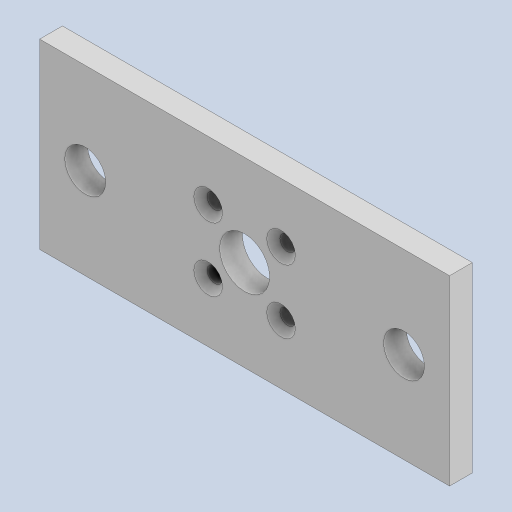
# Autodesk Inventor part: Al block2
Saved by Autodesk Inventor 2023.4 (Build 274418000, 418)
## iProperties
Created: 2024-01-11
Part Number: Al block2
Material: Generic
Document SubType Name: Modeling
Designer: PalumaCMM
Density: 1 g/cm^3
Appearance: Default
Author: PalumaCMM
Autodesk Inventor part; units mm, degrees
ref_plane "YZ Plane" through (0, 0, 0) normal (1, 0, 0) x (0, 1, 0)
ref_plane "XZ Plane" through (0, 0, 0) normal (0, 1, 0) x (-1, 0, 0)
ref_plane "XY Plane" through (0, 0, 0) normal (0, 0, 1) x (1, 0, 0)
sketch "Sketch1" plane through (0, 0, 0) normal (0, 0, 1) x (1, 0, 0)
  line L0 (0, 0) -> (60, 0)
  line L1 (60, 0) -> (60, 40)
  line L2 (60, 40) -> (0, 40)
  line L3 (0, 40) -> (0, 0)
  dimension "d0" = 60
  dimension "d1" = 40
  constraints: 8 end point, 2 parallel, 1 horizontal, 1 perpendicular
  measures "d0" distance of L2.end L1.end
  measures "d1" distance of L1.end L0.end
extrude "Extrusion1" add sketch "Sketch1" along normal blind 5
sketch "Sketch6" plane through (0, 0, 5) normal (0, 0, 1) x (1, 0, 0)
  point P0 (0, 0)
  point P1 (30, 20)
hole "Hole2" at (30, 20, 5) direction (0, 0, -1) diameter 11 end through all clearance for "Countersunk Flat Head Screw ISO 2009/7046" size "M10" standard "ISO"
sketch "Sketch7" plane through (0, 0, 5) normal (0, 0, 1) x (1, 0, 0)
  line L0 (0, 40) -> (0, 0) projected
  line L1 (60, 0) -> (60, 40) projected
  line L2 (60, 0) -> (0, 0)
  line L3 (60, 40) -> (0, 40) projected
  line L4 (30, 40) -> (30, 0)
  line L5 (0, 0) -> (60, 0) projected
  line L6 (0, 40) -> (0, 0) projected
  line L7 (0, 40) -> (-15, 40)
  line L8 (-15, 40) -> (-15, 0)
  line L9 (-15, 0) -> (0, 0)
  line L10 (0, 0) -> (0, 40)
  line L11 (60, 40) -> (60, 0)
  line L12 (60, 40) -> (60, 0)
  line L13 (60, 40) -> (75, 40)
  line L14 (75, 40) -> (75, 0)
  line L15 (75, 0) -> (60, 0)
  line L16 (0, 40) -> (-15, 40)
  point P0 (60, 0)
  point P1 (0, 0)
  dimension "d54" = 15
  dimension "d55" = 40
  constraints: 24 end point, 4 symmetric about line, 3 equal length, 2 midpoint, 2 point on line, 1 horizontal, 1 perpendicular
  measures "d54" distance of L9.end L8.end
  measures "d55" distance of L8.end L7.end
extrude "Extrusion3" add sketch "Sketch7" against normal blind 5 contours L0 L9 L8 L7 | L13 L14 L15 L1
sketch "Sketch9" plane through (0, 0, 5) normal (0, 0, 1) x (1, 0, 0)
  point P0 (0, 0)
  point P1 (-5, 20)
  point P2 (65, 20)
hole "Hole4" at (-5, 20, 5) at (65, 20, 5) direction (0, 0, -1) diameter 9 end through all clearance for "Countersunk Flat Head Screw ISO 2009/7046" size "M8" standard "ISO"
sketch "Sketch10" plane through (0, 0, 5) normal (0, 0, 1) x (1, 0, 0)
  line L0 (35.5, 14.5) -> (35.5, 25.5)
  line L1 (35.5, 14.5) -> (35.5, 25.5)
  line L2 (24.5, 25.5) -> (24.5, 14.5)
  line L3 (24.5, 25.5) -> (24.5, 14.5)
  line L4 (24.5, 14.5) -> (35.5, 25.5) construction
  line L5 (35.5, 14.5) -> (24.5, 25.5) construction
  circle A0 centre (30, 20) radius 5.5 projected
  line L6 (24.5, 30) -> (24.5, 10)
  line L7 (24.5, 10) -> (19.5, 10)
  line L8 (19.5, 10) -> (19.5, 30)
  line L9 (19.5, 30) -> (24.5, 30)
  line L10 (24.5, 20) -> (35.5, 20)
  line L11 (35.5, 30) -> (35.5, 10)
  line L12 (35.5, 10) -> (40.5, 10)
  line L13 (40.5, 10) -> (40.5, 30)
  line L14 (40.5, 30) -> (35.5, 30)
  point P0 (0, 0)
  point P1 (30, 25.5)
  point P2 (22, 13)
  point P3 (22, 27)
  point P4 (38, 13)
  point P5 (38, 27)
  dimension "d45" = 20
  dimension "d46" = 5
  constraints: 30 end point, 4 midpoint, 4 parallel, 3 point on circle, 1 perpendicular, 1 point on line
  measures "d45" distance of L7.end L8.end
  measures "d46" distance of L6.end L7.end
hole "Hole5" at (22, 13, 5) at (22, 27, 5) at (38, 13, 5) at (38, 27, 5) direction (0, 0, -1) diameter 3.4 end through all countersink diameter 6.3 countersink angle 90 clearance for "Countersunk Flat Head Screw ISO 2009/7046" size "M3" standard "ISO"
body "Solid1"
